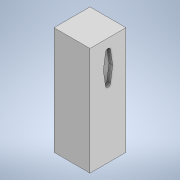
# Autodesk Inventor part: tangan kanan
Saved by Autodesk Inventor 2021 (Build 250183000, 183)
## iProperties
Created: 2025-04-02
Part Number: tangan kanan
Material: Generic
Document SubType Name: Modeling
Designer: Admin
Density: 1 g/cm^3
Appearance: Default
Author: Admin
Autodesk Inventor part; units mm, degrees
ref_plane "YZ Plane" through (0, 0, 0) normal (1, 0, 0) x (0, 1, 0)
ref_plane "XZ Plane" through (0, 0, 0) normal (0, 1, 0) x (-1, 0, 0)
ref_plane "XY Plane" through (0, 0, 0) normal (0, 0, 1) x (1, 0, 0)
sketch "Sketch1" plane through (0, 0, 0) normal (0, 1, 0) x (-1, 0, 0)
  line L0 (25, 25) -> (-25, 25)
  line L1 (-25, 25) -> (-25, -25)
  line L2 (-25, -25) -> (25, -25)
  line L3 (25, -25) -> (25, 25)
  line L4 (25, 25) -> (-25, -25) construction
  line L5 (-25, 25) -> (25, -25) construction
  point P0 (0, 0)
  dimension "d0" = 50
  dimension "d1" = 50
  constraints: 12 end point, 2 midpoint, 2 parallel, 1 horizontal, 1 perpendicular
  measures "d0" distance of L2.end L1.end
  measures "d1" distance of L1.end L0.end
extrude "Extrusion1" add sketch "Sketch1" along normal blind 150
sketch "Sketch2" plane through (25, 0, 25) normal (1, 0, 0) x (0, 0, -1)
  arc A0 (28.5, 134.119) -> (21.5, 134.119) centre (25, 134.119) ccw
  line L0 (31.5, 114.119) -> (28.5, 134.119)
  line L1 (21.5, 134.119) -> (18.5, 114.119)
  line L2 (25, 114.119) -> (27.6706, 114.119)
  arc A1 (21.5, 94.119) -> (28.5, 94.119) centre (25, 94.119) ccw
  line L3 (31.5, 114.119) -> (28.5, 94.119)
  line L4 (21.5, 94.119) -> (18.5, 114.119)
  arc A2 (18.7861, 116.0261) -> (18.7861, 112.2119) centre (25, 114.119) ccw
  arc A3 (31.2139, 112.2119) -> (31.2139, 116.0261) centre (25, 114.119) ccw
  point P0 (25, 0)
  dimension "d5" = 7
  dimension "d6" = 20
  constraints: 10 end point, 10 point on circle, 4 centre point, 4 point on line, 3 symmetric about line, 1 horizontal, 1 other
  measures "d5" diameter of A0
  measures "d6" distance of A0.centre L2.start
extrude "Extrusion2" cut sketch "Sketch2" against normal blind 5 contours L0 L3 A1 L4 L1 A0
body "Solid1"
